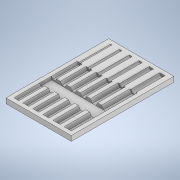
# Autodesk Inventor part: punchTray
Saved by Autodesk Inventor 2020.2 (Build 242310000, 310)
## iProperties
Created: 2019-12-07
Part Number: punchTray
Material: Generic
Document SubType Name: Modeling
Designer: robst
Density: 1 g/cm^3
Appearance: Default
Author: robst
Autodesk Inventor part; units mm, degrees
ref_plane "YZ Plane" through (0, 0, 0) normal (1, 0, 0) x (0, 1, 0)
ref_plane "XZ Plane" through (0, 0, 0) normal (0, 1, 0) x (-1, 0, 0)
ref_plane "XY Plane" through (0, 0, 0) normal (0, 0, 1) x (1, 0, 0)
sketch "Sketch3" plane through (0, 0, 0) normal (0, 0, 1) x (1, 0, 0)
  line L0 (-52.4636, -4.0957) -> (52.4636, -4.0957)
  line L1 (52.4636, -4.0957) -> (52.4636, 4.0958)
  line L2 (52.4636, 4.0958) -> (-52.4636, 4.0958)
  line L3 (-52.4636, 4.0958) -> (-52.4636, -4.0957)
  line L4 (-52.4636, -4.0957) -> (52.4636, 4.0958) construction
  line L5 (52.4636, -4.0957) -> (-52.4636, 4.0958) construction
  line L6 (46.1136, 4.0958) -> (43.2173, -0.9208)
  line L7 (43.2173, -0.9208) -> (37.4248, -0.9208)
  line L8 (37.4248, -0.9208) -> (34.5285, 4.0958)
  line L9 (34.5285, 4.0958) -> (37.4248, 9.1123)
  line L10 (37.4248, 9.1123) -> (43.2173, 9.1123)
  line L11 (43.2173, 9.1123) -> (46.1136, 4.0958)
  line L12 (28.1785, 4.0958) -> (25.2822, -0.9207)
  line L13 (25.2822, -0.9207) -> (19.4897, -0.9207)
  line L14 (19.4897, -0.9207) -> (16.5934, 4.0957)
  line L15 (16.5934, 4.0957) -> (19.4897, 9.1122)
  line L16 (19.4897, 9.1122) -> (25.2822, 9.1123)
  line L17 (25.2822, 9.1123) -> (28.1785, 4.0958)
  line L18 (0, 0) -> (0, 4.0957) construction
  line L19 (10.2434, 4.0958) -> (7.787, -0.1587)
  line L20 (7.787, -0.1587) -> (2.8744, -0.1587)
  line L21 (2.8744, -0.1587) -> (0.418, 4.0958)
  line L22 (0.418, 4.0958) -> (2.8744, 8.3503)
  line L23 (2.8744, 8.3503) -> (7.787, 8.3503)
  line L24 (7.787, 8.3503) -> (10.2434, 4.0958)
  line L25 (-5.932, 4.0958) -> (-8.3883, -0.1588)
  line L26 (-8.3883, -0.1588) -> (-13.301, -0.1587)
  line L27 (-13.301, -0.1587) -> (-15.7573, 4.0958)
  line L28 (-15.7573, 4.0958) -> (-13.301, 8.3503)
  line L29 (-13.301, 8.3503) -> (-8.3883, 8.3503)
  line L30 (-8.3883, 8.3503) -> (-5.932, 4.0958)
  line L31 (-22.1073, 4.0958) -> (-24.5416, -0.1206)
  line L32 (-24.5416, -0.1206) -> (-29.4103, -0.1206)
  line L33 (-29.4103, -0.1206) -> (-31.8447, 4.0958)
  line L34 (-31.8447, 4.0958) -> (-29.4103, 8.3122)
  line L35 (-29.4103, 8.3122) -> (-24.5416, 8.3122)
  line L36 (-24.5416, 8.3122) -> (-22.1073, 4.0958)
  line L37 (-38.1947, 4.0958) -> (-40.1744, 0.6668)
  line L38 (-40.1744, 0.6668) -> (-44.1339, 0.6668)
  line L39 (-44.1339, 0.6668) -> (-46.1136, 4.0958)
  line L40 (-46.1136, 4.0958) -> (-44.1339, 7.5248)
  line L41 (-44.1339, 7.5248) -> (-40.1744, 7.5247)
  line L42 (-40.1744, 7.5247) -> (-38.1947, 4.0958)
  point P0 (40.321, 4.0958)
  point P1 (22.3859, 4.0958)
  point P2 (34.5285, 4.0958)
  point P3 (16.5934, 4.0958)
  point P4 (5.3307, 4.0958)
  point P5 (-10.8446, 4.0958)
  point P6 (-26.976, 4.0958)
  point P7 (-42.1541, 4.0958)
  point P8 (0.418, 4.0958)
  point P9 (-15.7573, 4.0958)
  point P10 (-31.8447, 4.0958)
  point P11 (-46.1136, 4.0958)
  dimension "d7" = 10.033
  dimension "d8" = 10.033
  dimension "d13" = 6.35
  dimension "d14" = 6.35
  dimension "d15" = 8.509
  dimension "d16" = 6.35
  dimension "d17" = 8.509
  dimension "d18" = 6.35
  dimension "d19" = 8.4328
  dimension "d20" = 6.35
  dimension "d21" = 6.35
  dimension "d22" = 6.858
  dimension "d23" = 6.35
  dimension "d24" = 3.175
  constraints: 84 end point, 2 horizontal, 2 midpoint, 1 parallel, 1 perpendicular, 94 other
  measures "d7" distance between parallel lines of L7 L10
  measures "d8" distance between parallel lines of L13 L16
  measures "d13" distance of L6.start L1.end
  measures "d14" distance of L8.end L12.start
  measures "d15" distance between parallel lines of L20 L23
  measures "d16" distance of L14.end L19.start
  measures "d17" distance between parallel lines of L26 L29
  measures "d18" distance of L21.end L25.start
  measures "d19" distance between parallel lines of L32 L35
  measures "d20" distance of L27.end L31.start
  measures "d21" distance of L33.end L37.start
  measures "d22" distance between parallel lines of L38 L41
  measures "d23" distance from line of L39.end L3
  measures "d24" distance between parallel lines of L0 L7
extrude "Extrusion3" add sketch "Sketch3" against normal blind 152.4 contours L3 L2 L39 L38 L37 L33 L32 L31 L27 L26 L25 L21 L20 L19 L14 L13 L12 L8 L7 L6 L1 L0
sketch "Sketch4" plane through (0, 0, 0) normal (0, 0, 1) x (1, 0, 0)
  line L0 (52.4636, -4.0957) -> (-52.4636, -4.0957) projected
  line L1 (52.4636, 4.0958) -> (52.4636, -4.0957) projected
  line L2 (-52.4636, -4.0957) -> (52.4636, -4.0957)
  line L3 (52.4636, -4.0957) -> (52.4636, 4.0958)
  line L4 (52.4636, 4.0958) -> (-52.4636, 4.0957)
  line L5 (-52.4636, 4.0957) -> (-52.4636, -4.0957)
  point P0 (0, 0)
  constraints: 8 end point, 2 parallel, 1 horizontal, 1 perpendicular
extrude "Extrusion4" add sketch "Sketch4" along normal blind 6.35
sketch "Sketch6" plane through (0, 0, -152.4) normal (0, 0, -1) x (-1, 0, 0)
  line L0 (-37.4248, -0.9208) -> (-43.2173, -0.9208) construction
  line L1 (-40.321, -0.9208) -> (-40.321, 4.0958) construction
  line L2 (-52.4636, 4.0958) -> (52.4636, 4.0957) construction
  arc A0 (-44.5438, 4.0958) -> (-36.0983, 4.0958) centre (-40.321, 4.0958) ccw
  line L3 (-34.5285, 4.0958) -> (-37.4248, -0.9208)
  line L4 (-37.4248, -0.9208) -> (-43.2173, -0.9208)
  line L5 (-43.2173, -0.9208) -> (-46.1136, 4.0958)
  line L6 (-46.1136, 4.0958) -> (-44.5438, 4.0958)
  line L7 (-34.5285, 4.0958) -> (-36.0983, 4.0958)
  point P0 (0, 0)
  dimension "d31" = 8.4455
  constraints: 12 end point, 3 point on line, 2 coincident, 2 point on circle, 1 centre point, 1 midpoint, 1 vertical, 6 other
  measures "d31" diameter of A0
extrude "5_16_punch" add sketch "Sketch6" against normal blind 46.355
sketch "Sketch7" plane through (0, 0, -152.4) normal (0, 0, -1) x (-1, 0, 0)
  line L0 (-28.1785, 4.0958) -> (-16.5934, 4.0958) projected
  line L1 (-16.5934, 4.0958) -> (-19.4897, -0.9207)
  line L2 (-19.4897, -0.9207) -> (-25.2822, -0.9207)
  line L3 (-25.2822, -0.9207) -> (-28.1785, 4.0958)
  arc A0 (-25.8149, 4.0958) -> (-18.9569, 4.0958) centre (-22.3859, 4.0958) ccw
  line L4 (-28.1785, 4.0958) -> (-25.8149, 4.0958)
  line L5 (-10.2434, 4.0958) -> (-16.5934, 4.0958) projected
  line L6 (-16.5934, 4.0958) -> (-18.9569, 4.0958)
  point P0 (0, 0)
  dimension "d34" = 6.858
  constraints: 10 end point, 2 point on circle, 2 point on line, 1 centre point, 1 coincident, 1 midpoint, 6 other
  measures "d34" diameter of A0
extrude "1_4_punch" add sketch "Sketch7" against normal blind 47.625 contours L0 A0 L1 L2 L3
sketch "Sketch8" plane through (0, 0, -152.4) normal (0, 0, -1) x (-1, 0, 0)
  line L0 (-10.2434, 4.0958) -> (-0.418, 4.0958) projected
  line L1 (-0.418, 4.0958) -> (-2.8744, -0.1588)
  line L2 (-2.8744, -0.1588) -> (-7.787, -0.1587)
  line L3 (-7.787, -0.1587) -> (-10.2434, 4.0958)
  arc A0 (-7.966, 4.0958) -> (-2.6955, 4.0958) centre (-5.3307, 4.0958) ccw
  line L4 (-10.2434, 4.0958) -> (-7.787, -0.1587) projected
  line L5 (-10.2434, 4.0958) -> (-7.966, 4.0958)
  line L6 (-0.418, 4.0958) -> (-2.6955, 4.0958)
  point P0 (0, 0)
  point P1 (-10.2434, 4.0958)
  dimension "d37" = 5.2705
  constraints: 10 end point, 2 point on circle, 2 point on line, 1 centre point, 1 coincident, 1 midpoint, 6 other
  measures "d37" diameter of A0
extrude "3_16_punch" add sketch "Sketch8" against normal blind 50.8 contours L0 A0 L1 L2 L3
sketch "Sketch9" plane through (0, 0, -152.4) normal (0, 0, -1) x (-1, 0, 0)
  line L0 (13.301, -0.1587) -> (8.3883, -0.1588) construction
  line L1 (10.8446, -0.1587) -> (10.8446, 4.0957) construction
  line L2 (-52.4636, 4.0958) -> (52.4636, 4.0957) construction
  line L3 (15.7573, 4.0958) -> (13.301, -0.1587) projected
  line L4 (15.7573, 4.0958) -> (13.301, -0.1588)
  line L5 (13.301, -0.1588) -> (8.3883, -0.1588)
  line L6 (8.3883, -0.1588) -> (5.932, 4.0958)
  arc A0 (8.6063, 4.0957) -> (13.083, 4.0957) centre (10.8446, 4.0957) ccw
  line L7 (8.3883, -0.1588) -> (5.932, 4.0958) projected
  line L8 (5.932, 4.0958) -> (8.6063, 4.0957)
  line L9 (22.1073, 4.0958) -> (15.7573, 4.0958) projected
  line L10 (15.7573, 4.0958) -> (13.083, 4.0957)
  point P0 (0, 0)
  point P1 (13.301, -0.1588)
  dimension "d40" = 4.4768
  constraints: 12 end point, 3 point on line, 2 coincident, 2 point on circle, 1 centre point, 1 midpoint, 1 vertical, 6 other
  measures "d40" diameter of A0
extrude "5_32_punch" add sketch "Sketch9" against normal blind 50.8
sketch "Sketch11" plane through (0, 0, -152.4) normal (0, 0, -1) x (-1, 0, 0)
  line L0 (22.1073, 4.0958) -> (31.8447, 4.0958) projected
  line L1 (29.4103, -0.1206) -> (31.8447, 4.0958) projected
  line L2 (31.8447, 4.0958) -> (29.4103, -0.1206)
  line L3 (29.4103, -0.1206) -> (24.5416, -0.1206)
  line L4 (24.5416, -0.1206) -> (22.1073, 4.0958)
  arc A0 (25.1345, 4.0958) -> (28.8175, 4.0958) centre (26.976, 4.0958) ccw
  line L5 (22.1073, 4.0958) -> (24.5416, -0.1206) projected
  line L6 (22.1073, 4.0958) -> (25.1345, 4.0958)
  line L7 (31.8447, 4.0958) -> (28.8175, 4.0958)
  point P0 (0, 0)
  point P1 (29.4103, -0.1206)
  dimension "d44" = 3.683
  constraints: 10 end point, 2 point on circle, 2 point on line, 1 centre point, 1 coincident, 1 midpoint, 6 other
  measures "d44" diameter of A0
extrude "1_8_punch" add sketch "Sketch11" against normal blind 50.8 contours L0 A0 L1 L3 L4
sketch "Sketch12" plane through (0, 0, -152.4) normal (0, 0, -1) x (-1, 0, 0)
  line L0 (40.1744, 0.6668) -> (44.1339, 0.6668) construction
  line L1 (42.1541, 0.6668) -> (42.1541, 4.0957) construction
  line L2 (-52.4636, 4.0958) -> (52.4636, 4.0957) construction
  line L3 (44.1339, 0.6668) -> (46.1136, 4.0958) projected
  line L4 (46.1136, 4.0958) -> (44.1339, 0.6668)
  line L5 (44.1339, 0.6668) -> (40.1744, 0.6667)
  line L6 (40.1744, 0.6667) -> (38.1947, 4.0958)
  arc A0 (41.1064, 4.0957) -> (43.2019, 4.0957) centre (42.1541, 4.0957) ccw
  line L7 (38.1947, 4.0958) -> (28.8175, 4.0958) projected
  line L8 (38.1947, 4.0958) -> (41.1064, 4.0957)
  line L9 (46.1136, 4.0958) -> (43.2019, 4.0957)
  point P0 (0, 0)
  point P1 (44.1339, 0.6668)
  dimension "d47" = 2.0955
  constraints: 12 end point, 3 point on line, 2 coincident, 2 point on circle, 1 centre point, 1 midpoint, 1 vertical, 6 other
  measures "d47" diameter of A0
extrude "1_16_punch" add sketch "Sketch12" against normal blind 50.8
sketch "Sketch5" plane through (0, 0, -152.4) normal (0, 0, -1) x (-1, 0, 0)
  line L0 (-52.4636, 4.0958) -> (-52.4636, -4.0957) projected
  line L1 (52.4636, 4.0958) -> (46.1136, 4.0958) projected
  line L2 (-52.4636, -4.0957) -> (52.4636, -4.0957)
  line L3 (52.4636, -4.0957) -> (52.4636, 4.0958)
  line L4 (52.4636, 4.0958) -> (-52.4636, 4.0957)
  line L5 (-52.4636, 4.0957) -> (-52.4636, -4.0957)
  point P0 (0, 0)
  point P1 (-52.4636, 4.0957)
  constraints: 8 end point, 2 parallel, 1 horizontal, 1 perpendicular
extrude "Extrusion5" add sketch "Sketch5" along normal blind 6.35
sketch "Sketch13" plane through (-52.4636, 4.0958, 6.35) normal (0, 1, 0) x (1, 0, 0)
  line L0 (6.35, 6.35) -> (6.35, 107.95) projected
  line L1 (98.5772, 6.35) -> (98.5772, 112.395) projected
  line L2 (6.35, 47.625) -> (98.5772, 47.625)
  line L3 (98.5772, 47.625) -> (98.5772, 66.675)
  line L4 (98.5772, 66.675) -> (6.35, 66.675)
  line L5 (6.35, 66.675) -> (6.35, 47.625)
  line L6 (6.35, 57.15) -> (98.5772, 57.15) construction
  line L7 (14.2689, 6.35) -> (6.35, 6.35) construction
  point P0 (52.4636, 6.35)
  point P1 (6.35, 66.675)
  dimension "d50" = 19.05
  dimension "d51" = 50.8
  constraints: 10 end point, 2 midpoint, 2 parallel, 2 point on line, 1 horizontal, 1 perpendicular
  measures "d50" distance between parallel lines of L4 L2
  measures "d51" distance between parallel lines of L6 L7
extrude "Extrusion12" cut sketch "Sketch13" against normal blind 5.08
equation "\"d14\" = gapBetweenParts"
equation "\"d16\" = gapBetweenParts"
equation "\"d18\" = gapBetweenParts"
equation "\"d20\" = gapBetweenParts"
equation "\"d21\" = gapBetweenParts"
equation "\"gapBetweenParts\" = 6.35"
body "Solid3"
